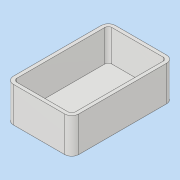
# Autodesk Inventor part: BatteryCaseSide1
Saved by Autodesk Inventor 2017 (Build 210142000, 142)
## iProperties
Created: 2018-02-14
Part Number: BatteryCaseSide1
Material: ABS Plastic
Document SubType Name: Modeling
Designer: Derek Wider
Density: 1.06 g/cm^3
Appearance: Smooth - White
Author: Derek Wider
Autodesk Inventor part; units mm, degrees
ref_plane "YZ Plane" through (0, 0, 0) normal (1, 0, 0) x (0, 1, 0)
ref_plane "XZ Plane" through (0, 0, 0) normal (0, 1, 0) x (-1, 0, 0)
ref_plane "XY Plane" through (0, 0, 0) normal (0, 0, 1) x (1, 0, 0)
sketch "Sketch1" plane through (0, 0, 0) normal (0, 1, 0) x (-1, 0, 0)
  line L0 (4.7625, 0) -> (51.1175, 0)
  line L1 (55.88, -4.7625) -> (55.88, -84.1375)
  line L2 (51.1175, -88.9) -> (4.7625, -88.9)
  line L3 (0, -84.1375) -> (0, -4.7625)
  arc A0 (55.88, -4.7625) -> (51.1175, 0) centre (51.1175, -4.7625) ccw
  arc A1 (4.7625, 0) -> (0, -4.7625) centre (4.7625, -4.7625) ccw
  arc A2 (0, -84.1375) -> (4.7625, -88.9) centre (4.7625, -84.1375) ccw
  arc A3 (51.1175, -88.9) -> (55.88, -84.1375) centre (51.1175, -84.1375) ccw
  line L4 (54.2925, -84.1375) -> (54.2925, -4.7625)
  arc A4 (54.2925, -4.7625) -> (51.1175, -1.5875) centre (51.1175, -4.7625) ccw
  line L5 (51.1175, -1.5875) -> (4.7625, -1.5875)
  arc A5 (4.7625, -1.5875) -> (1.5875, -4.7625) centre (4.7625, -4.7625) ccw
  line L6 (1.5875, -4.7625) -> (1.5875, -84.1375)
  arc A6 (1.5875, -84.1375) -> (4.7625, -87.3125) centre (4.7625, -84.1375) ccw
  line L7 (4.7625, -87.3125) -> (51.1175, -87.3125)
  arc A7 (51.1175, -87.3125) -> (54.2925, -84.1375) centre (51.1175, -84.1375) ccw
  line L8 (57.4675, -84.1375) -> (57.4675, -4.7625)
  arc A8 (57.4675, -4.7625) -> (51.1175, 1.5875) centre (51.1175, -4.7625) ccw
  line L9 (51.1175, 1.5875) -> (4.7625, 1.5875)
  arc A9 (4.7625, 1.5875) -> (-1.5875, -4.7625) centre (4.7625, -4.7625) ccw
  line L10 (-1.5875, -4.7625) -> (-1.5875, -84.1375)
  arc A10 (-1.5875, -84.1375) -> (4.7625, -90.4875) centre (4.7625, -84.1375) ccw
  line L11 (4.7625, -90.4875) -> (51.1175, -90.4875)
  arc A11 (51.1175, -90.4875) -> (57.4675, -84.1375) centre (51.1175, -84.1375) ccw
  point P0 (0, 0)
  point P1 (55.88, -88.9)
  point P2 (55.88, 0)
  point P3 (0, -88.9)
  dimension "d0" = 88.9
  dimension "d1" = 55.88
  dimension "d2" = 4.7625
  dimension "d3" = 1.5875
  dimension "d4" = 1.5875
  constraints: 24 end point, 24 point on circle, 12 centre point, 8 point on line, 8 tangent, 6 parallel, 3 equal radius, 3 perpendicular, 1 horizontal, 14 other
  measures "d0" distance of point (55.88, 0) point (55.88, -88.9)
  measures "d1" distance of point (55.88, -88.9) point (0, -88.9)
  measures "d2" radius of A0
  measures "d3" distance between parallel lines of L1 L4
  measures "d4" distance between parallel lines of L1 L8
extrude "Extrusion1" add sketch "Sketch1" along normal blind 31.75 contours L0 A0 L1 A3 L2 A2 L3 A1 | A11 L11 A10 L10 A9 L9 A8 L8
extrude "Extrusion2" add sketch "Sketch1" along normal blind 3.175 contours A7 L7 A6 L6 A5 L5 A4 L4
equation "\"d3\" = d4"
body "Solid1"
